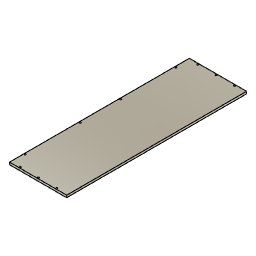
side_cover_lid v28 (Autodesk Fusion 360 design; units mm, degrees)
Autodesk Fusion 360 part; units mm, degrees
sketch "Sketch4" plane through (0, 0, 0) normal (1, 0, 0) x (0, 1, 0)
  line L0 (0, 0) -> (-450, 0)
  line L1 (-450, 0) -> (-450, 170.719)
  line L2 (-450, 170.719) -> (0, 170.719)
  line L3 (0, 170.719) -> (0, 0)
  dimension "d21" = 450
  dimension "d22" = 170.719
  constraint horizontal L0
  constraint vertical L1
  constraint horizontal L2
  constraint vertical L3
  constraint coincident L0.start L3.end
  measures "d21" distance of L0.start L0.end
  measures "d22" distance of L0.start L2.end
sketch "Sketch5" plane through (0, 0, 0) normal (-1, 0, 0) x (0, -1, 0)
  line L0 (450, 170.719) -> (0, 170.719)
  line L1 (0, 170.719) -> (0, 0)
  line L2 (0, 0) -> (450, 0)
  line L3 (450, 0) -> (450, 170.719)
  line L4 (0, 170.719) -> (455, 170.719)
  line L5 (455, 170.719) -> (455, 175.719)
  line L6 (455, 175.719) -> (0, 175.719)
  line L7 (0, 175.719) -> (0, 170.719)
  line L8 (455, 175.719) -> (450, 175.719)
  line L9 (450, 175.719) -> (450, 0)
  line L10 (450, 0) -> (455, 0)
  line L11 (455, 0) -> (455, 175.719)
  line L12 (0, 0) -> (-5, 0)
  line L13 (-5, 0) -> (-5, 175.719)
  line L14 (-5, 175.719) -> (0, 175.719)
  line L15 (0, 175.719) -> (0, 0)
  dimension "d25" = 455
  dimension "d26" = 5
  dimension "d27" = 5
  dimension "d28" = 175.719
  constraint horizontal L4
  constraint vertical L5
  constraint horizontal L6
  constraint vertical L7
  constraint coincident L0.end L1.start
  constraint horizontal L8
  constraint vertical L9
  constraint horizontal L10
  constraint vertical L11
  constraint coincident L2.end L3.start
  constraint horizontal L12
  constraint vertical L13
  constraint horizontal L14
  constraint vertical L15
  constraint coincident L1.end L2.start
  measures "d25" distance of L0.end L4.end
  measures "d26" distance of L0.end L6.end
  measures "d27" distance of L1.end L12.end
  measures "d28" distance of L1.end L6.end
extrude "Extrude7" add sketch "Sketch5" along normal blind 150 contours L3 L4 L9 L10 L11 | L0 L4 L6 L7 L9 L15 | L1 L7 L12 L13 L14 L15
extrude "Extrude8" add 1 faces at (-50, -451.6667, 170.719) along direction (0, 0, 1) blind 5
sketch "Sketch6" plane through (0, 0, 0) normal (1, 0, 0) x (0, 1, 0)
  line L0 (-450, 0) -> (-450, 170.719)
  line L1 (-450, 170.719) -> (0, 170.719)
  line L2 (0, 170.719) -> (0, 0)
  line L3 (0, 0) -> (5, 0)
  line L4 (5, 0) -> (5, 175.719)
  line L5 (5, 175.719) -> (-455, 175.719)
  line L6 (-455, 175.719) -> (-455, 0)
  line L7 (-455, 0) -> (-450, 0)
  line L8 (-455, 175.719) -> (5, 175.719)
  line L9 (5, 175.719) -> (5, 0)
  line L10 (5, 0) -> (-455, 0)
  line L11 (-455, 0) -> (-455, 175.719)
  constraint horizontal L8
  constraint vertical L9
  constraint horizontal L10
  constraint vertical L11
  constraint coincident L3.end L4.start
  constraint coincident L5.end L6.start
extrude "Extrude9" add sketch "Sketch6" along normal blind 5
sketch "Sketch7" plane through (0, -455, 0) normal (0, -1, 0) x (1, 0, 0)
  line L0 (5, 175.719) -> (-150, 175.719)
  line L1 (-150, 175.719) -> (-150, 0)
  line L2 (-150, 0) -> (5, 0)
  line L3 (5, 0) -> (5, 175.719)
  line L4 (-150, 0) -> (5, 0)
  line L5 (5, 0) -> (5, 5)
  line L6 (5, 5) -> (-150, 5)
  line L7 (-150, 5) -> (-150, 0)
  dimension "d35" = 5
  constraint horizontal L4
  constraint vertical L5
  constraint horizontal L6
  constraint vertical L7
  constraint coincident L3 L5.end
  constraint coincident L1.end L2.start
  measures "d35" distance of L1.end L6.end
extrude "Extrude10" add sketch "Sketch7" along normal blind 20 contours L1 L2 L3 L4 L5 L6 L7
sketch "Sketch8" plane through (0, 5, 0) normal (0, 1, 0) x (-1, 0, 0)
  line L0 (-5, 0) -> (150, 0)
  line L1 (150, 0) -> (150, 175.719)
  line L2 (150, 175.719) -> (-5, 175.719)
  line L3 (-5, 175.719) -> (-5, 0)
  line L4 (150, 0) -> (-5, 0)
  line L5 (-5, 0) -> (-5, 5)
  line L6 (-5, 5) -> (150, 5)
  line L7 (150, 5) -> (150, 0)
  dimension "d38" = 5
  constraint horizontal L4
  constraint vertical L5
  constraint horizontal L6
  constraint vertical L7
  constraint coincident L3 L5.end
  constraint coincident L0.end L1.start
  measures "d38" distance of L0.end L6.end
extrude "Extrude11" add sketch "Sketch8" along normal blind 20 contours L0 L1 L3 L4 L5 L6 L7
sketch "Sketch9" plane through (5, 0, 0) normal (1, 0, 0) x (0, 1, 0)
  line L0 (-475, 0) -> (25, 0)
  line L1 (25, 0) -> (25, 5)
  line L2 (25, 5) -> (5, 5)
  line L3 (5, 5) -> (5, 175.719)
  line L4 (5, 175.719) -> (-455, 175.719)
  line L5 (-455, 175.719) -> (-455, 5)
  line L6 (-455, 5) -> (-475, 5)
  line L7 (-475, 5) -> (-475, 0)
  line L8 (-475, 5) -> (25, 5)
  line L9 (25, 5) -> (25, 0)
  line L10 (25, 0) -> (-475, 0)
  line L11 (-475, 0) -> (-475, 5)
  constraint horizontal L8
  constraint vertical L9
  constraint horizontal L10
  constraint vertical L11
  constraint coincident L0.end L1.start
  constraint coincident L6.end L7.start
extrude "Extrude12" add sketch "Sketch9" along normal blind 20 contours L0 L1 L2 L6 L7 L8 L9 L10 L11
sketch "Sketch10" plane through (0, 0, 5) normal (0, 0, 1) x (-1, 0, 0)
  line L0 (150, -5) -> (-5, -5)
  line L1 (-5, -5) -> (-5, 455)
  line L2 (-5, 455) -> (150, 455)
  line L3 (150, 455) -> (150, 475)
  line L4 (150, 475) -> (-25, 475)
  line L5 (-25, 475) -> (-25, -25)
  line L6 (-25, -25) -> (150, -25)
  line L7 (150, -25) -> (150, -5)
  line L8 (-25, -25) -> (-5, -25)
  line L9 (-5, -25) -> (-5, -5)
  line L10 (-5, -5) -> (-25, -5)
  line L11 (-25, -5) -> (-25, -25)
  line L12 (-25, 475) -> (-5, 475)
  line L13 (-5, 475) -> (-5, 455)
  line L14 (-5, 455) -> (-25, 455)
  line L15 (-25, 455) -> (-25, 475)
  constraint horizontal L8
  constraint vertical L9
  constraint horizontal L10
  constraint vertical L11
  constraint coincident L0.end L1.start
  constraint coincident L5.end L6.start
  constraint horizontal L12
  constraint vertical L13
  constraint horizontal L14
  constraint vertical L15
  constraint coincident L1.end L2.start
  constraint coincident L4.end L5.start
extrude "Extrude13" cut sketch "Sketch10" against normal blind 50 contours L5 L6 L8 L9 L10 L11 | L4 L5 L12 L13 L14 L15
sketch "Sketch11" plane through (0, 0, 5) normal (0, 0, 1) x (-1, 0, 0)
  line L0 (-5, 475) -> (-5, 455)
  line L1 (-5, 455) -> (150, 455)
  line L2 (150, 455) -> (150, 475)
  line L3 (150, 475) -> (-5, 475)
  line L4 (-5, -25) -> (15, -25)
  line L5 (15, -25) -> (15, -15)
  line L6 (15, -15) -> (-5, -15)
  line L7 (-5, -15) -> (-5, -25)
  line L8 (150, -25) -> (130, -25)
  line L9 (130, -25) -> (130, -15)
  line L10 (130, -15) -> (150, -15)
  line L11 (150, -15) -> (150, -25)
  line L12 (130, -15) -> (72.5, -15)
  line L13 (150, 475) -> (130, 475)
  line L14 (130, 475) -> (130, 465)
  line L15 (130, 465) -> (150, 465)
  line L16 (150, 465) -> (150, 475)
  line L17 (-5, 475) -> (15, 475)
  line L18 (15, 475) -> (15, 465)
  line L19 (15, 465) -> (-5, 465)
  line L20 (-5, 465) -> (-5, 475)
  line L21 (130, 465) -> (72.5, 465)
  line L22 (-5, 455) -> (-15, 455)
  line L23 (-15, 455) -> (-15, 435)
  line L24 (-15, 435) -> (-5, 435)
  line L25 (-5, 435) -> (-5, 455)
  line L26 (-5, -5) -> (-15, -5)
  line L27 (-15, -5) -> (-15, 15)
  line L28 (-15, 15) -> (-5, 15)
  line L29 (-5, 15) -> (-5, -5)
  line L30 (-15, 15) -> (-15, 99)
  line L31 (-15, 99) -> (-15, 183)
  line L32 (-15, 183) -> (-15, 267)
  line L33 (-15, 267) -> (-15, 351)
  line L34 (-15, 351) -> (-15, 435)
  dimension "d45" = 20
  dimension "d46" = 10
  dimension "d47" = 20
  dimension "d48" = 10
  dimension "d49" = 57.5
  dimension "d50" = 20
  dimension "d51" = 20
  dimension "d52" = 57.5
  dimension "d53" = 10
  dimension "d54" = 20
  dimension "d55" = 10
  dimension "d56" = 20
  dimension "d57" = 84
  dimension "d58" = 84
  dimension "d59" = 84
  dimension "d60" = 84
  dimension "d61" = 84
  constraint horizontal L4
  constraint vertical L5
  constraint horizontal L6
  constraint vertical L7
  constraint horizontal L8
  constraint vertical L9
  constraint horizontal L10
  constraint vertical L11
  constraint perpendicular L9 L12
  constraint horizontal L13
  constraint vertical L14
  constraint horizontal L15
  constraint vertical L16
  constraint coincident L2.end L3.start
  constraint horizontal L17
  constraint vertical L18
  constraint horizontal L19
  constraint vertical L20
  constraint coincident L0.start L3.end
  constraint perpendicular L14 L21
  constraint horizontal L22
  constraint vertical L23
  constraint horizontal L24
  constraint vertical L25
  constraint coincident L0.end L1.start
  constraint horizontal L26
  constraint vertical L27
  constraint horizontal L28
  constraint vertical L29
  constraint perpendicular L28 L30
  constraint parallel L30 L31
  constraint parallel L31 L32
  constraint parallel L32 L33
  constraint vertical L34
  measures "d45" distance of L4.start L4.end
  measures "d46" distance of L4.start L6.end
  measures "d47" distance of L8.start L8.end
  measures "d48" distance of L8.start L10.end
  measures "d49" distance of L9.end L12.end
  measures "d50" distance of L2.end L13.end
  measures "d51" distance of L0.start L17.end
  measures "d52" distance of L14.end L21.end
  measures "d53" distance of L0.end L22.end
  measures "d54" distance of L0.end L24.end
  measures "d55" distance of L26.start L26.end
  measures "d56" distance of L26.start L28.end
  measures "d57" distance of L27.end L30.end
  measures "d58" distance of L30.end L31.end
  measures "d59" distance of L31.end L32.end
  measures "d60" distance of L32.end L33.end
  measures "d61" distance of L33.end L23.end
hole "Hole1" at (-130, -465, 5) at (-72.5, -465, 5) at (-15, -465, 5) at (15, -435, 5) at (15, -351, 5) at (15, -267, 5) at (15, -183, 5) at (15, -99, 5) at (15, -15, 5) at (-15, 15, 5) at (-72.5, 15, 5) at (-130, 15, 5) direction (0, 0, -1) diameter 7.035 depth 10 tip angle 180
thread "Thread1" "ISO Metric profile 8.0 M8x1 6H"
extrude "Extrude14" add 1 faces at (-98.3333, -148.3333, 175.719) along direction (0, 0, 1) blind 5
extrude "Extrude15" add 1 faces at (-46.6667, 5, 122.146) along direction (0, 1, 0) blind 5
extrude "Extrude16" add 1 faces at (-46.6667, -455, 122.146) along direction (0, -1, 0) blind 5
extrude "Extrude17" add 1 faces at (-144.4764, -463.0724, 0) along direction (0, 0, -1) blind 5
extrude "Extrude18" add 1 faces at (-46.6667, 25, -1.6667) along direction (0, 1, 0) blind 5
extrude "Extrude19" add 1 faces at (-46.6667, -475, -1.6667) along direction (0, -1, 0) blind 5
extrude "Extrude20" add 1 faces at (25, -301.6667, 1.6667) along direction (1, 0, 0) blind 5
extrude "Extrude21" add 1 faces at (21.6667, -455, 1.6667) along direction (0, -1, 0) blind 25
extrude "Extrude22" add 1 faces at (21.6667, 5, 1.6667) along direction (0, 1, 0) blind 25
sketch "Sketch12" plane through (0, 0, 5) normal (0, 0, 1) x (-1, 0, 0)
  circle A0 centre (72.5, 465) radius 3.5175
  circle A1 centre (130, 465) radius 3.5175
  circle A2 centre (15, 465) radius 3.5175
  circle A3 centre (-15, 15) radius 3.5175
  circle A4 centre (-15, 183) radius 3.5175
  circle A5 centre (-15, 351) radius 3.5175
  circle A6 centre (-15, 435) radius 3.5175
  circle A7 centre (-15, 267) radius 3.5175
  circle A8 centre (-15, 99) radius 3.5175
  line L0 (150, -10) -> (-5, -10)
  line L1 (-5, -10) -> (-5, 460)
  line L2 (-5, 460) -> (150, 460)
  line L3 (150, 460) -> (150, 480)
  line L4 (150, 480) -> (-30, 480)
  line L5 (-30, 480) -> (-30, -30)
  line L6 (-30, -30) -> (150, -30)
  line L7 (150, -30) -> (150, -10)
  circle A9 centre (72.5, -15) radius 3.5175
  circle A10 centre (15, -15) radius 3.5175
  circle A11 centre (130, -15) radius 3.5175
  line L8 (130, -15) -> (130, -20)
  line L9 (130, 465) -> (130, 470)
  line L10 (72.5, 465) -> (72.5, 470)
  line L11 (15, 465) -> (15, 470)
  line L12 (-15, 435) -> (-20, 435)
  line L13 (-15, 351) -> (-20, 351)
  line L14 (-15, 267) -> (-20, 267)
  line L15 (-15, 183) -> (-20, 183)
  line L16 (72.5, -15) -> (72.5, -20)
  line L17 (15, -15) -> (15, -20)
  line L18 (-15, 15) -> (-20, 15)
  line L19 (-15, 99) -> (-20, 99)
  dimension "d83" = 5
  dimension "d84" = 5
  dimension "d85" = 5
  dimension "d86" = 5
  dimension "d87" = 5
  dimension "d88" = 5
  dimension "d89" = 5
  dimension "d90" = 5
  dimension "d91" = 5
  dimension "d92" = 5
  dimension "d93" = 5
  dimension "d94" = 5
  constraint coincident A11.centre L8.start
  constraint perpendicular L6 L8
  constraint coincident A1.centre L9.start
  constraint perpendicular L2 L9
  constraint coincident A0.centre L10.start
  constraint perpendicular L2 L10
  constraint coincident A2.centre L11.start
  constraint perpendicular L4 L11
  constraint coincident A6.centre L12.start
  constraint horizontal L12
  constraint coincident A5.centre L13.start
  constraint perpendicular L5 L13
  constraint coincident A7.centre L14.start
  constraint perpendicular L1 L14
  constraint coincident A4.centre L15.start
  constraint perpendicular L1 L15
  constraint coincident A9.centre L16.start
  constraint perpendicular L0 L16
  constraint coincident A10.centre L17.start
  constraint perpendicular L0 L17
  constraint coincident A3.centre L18.start
  constraint horizontal L18
  constraint coincident A8.centre L19.start
  constraint perpendicular L5 L19
  measures "d83" distance of A11.centre L8.end
  measures "d84" distance of A1.centre L9.end
  measures "d85" distance of A0.centre L10.end
  measures "d86" distance of A2.centre L11.end
  measures "d87" distance of A6.centre L12.end
  measures "d88" distance of A5.centre L13.end
  measures "d89" distance of A7.centre L14.end
  measures "d90" distance of A4.centre L15.end
  measures "d91" distance of A9.centre L16.end
  measures "d92" distance of A10.centre L17.end
  measures "d93" distance of A3.centre L18.end
  measures "d94" distance of A8.centre L19.end
delete_face "DeleteFace1" 1 faces at (15.1753, -18.5131, -1.6667)
delete_face "DeleteFace2" 1 faces at (-14.8247, 11.4869, -1.6667)
delete_face "DeleteFace3" 1 faces at (-71.2969, 18.3054, -1.6667)
delete_face "DeleteFace4" 1 faces at (-129.8247, 11.4869, -1.6667)
delete_face "DeleteFace5" 1 faces at (15.1753, -102.5131, -1.6667)
delete_face "DeleteFace6" 1 faces at (-133.5164, -464.9123, -1.6667)
delete_face "DeleteFace7" 1 faces at (-76.0164, -464.9123, -1.6667)
delete_face "DeleteFace8" 1 faces at (-18.5164, -464.9123, -1.6667)
delete_face "DeleteFace9" 1 faces at (11.4836, -434.9123, -1.6667)
delete_face "DeleteFace10" 1 faces at (11.4836, -350.9123, -1.6667)
delete_face "DeleteFace11" 1 faces at (11.4836, -266.9123, -1.6667)
delete_face "DeleteFace12" 1 faces at (17.261, -180.3054, -1.6667)
hole "Hole2" at (-130, 20, 5) at (-72.5, 20, 5) at (-15, 20, 5) at (20, -15, 5) at (20, -99, 5) at (20, -183, 5) at (20, -267, 5) at (20, -351, 5) at (20, -435, 5) at (-15, -470, 5) at (-72.5, -470, 5) at (-130, -470, 5) direction (0, 0, -1) diameter 7.035 depth 38 tip angle 180
thread "Thread2" "ISO Metric profile 8.0 M8x1 6H"
extrude "Extrude23" add 1 faces at (-50, -300, 170.719) along direction (0, 0, -1) blind 43
extrude "Extrude24" cut 1 faces at (-98.3333, -303.3333, 180.719) along direction (0, 0, -1) blind 43
extrude "Extrude25" cut 1 faces at (30, -140, -1.6667) along direction (-1, 0, 0) blind 5
sketch "Sketch13" plane through (0, 0, 5) normal (0, 0, 1) x (-1, 0, 0)
  line L0 (-25, 480) -> (-25, -30)
  line L1 (-25, -30) -> (150, -30)
  line L2 (150, -30) -> (150, -10)
  line L3 (150, -10) -> (-5, -10)
  line L4 (-5, -10) -> (-5, 460)
  line L5 (-5, 460) -> (150, 460)
  line L6 (150, 460) -> (150, 480)
  line L7 (150, 480) -> (-25, 480)
  circle A0 centre (72.5, 470) radius 3.5175
  circle A1 centre (-20, 435) radius 3.5175
  circle A2 centre (-20, 267) radius 3.5175
  circle A3 centre (-20, 99) radius 3.5175
  circle A4 centre (15, -20) radius 3.5175
  circle A5 centre (130, -20) radius 3.5175
  circle A6 centre (72.5, -20) radius 3.5175
  circle A7 centre (-20, 15) radius 3.5175
  circle A8 centre (-20, 183) radius 3.5175
  circle A9 centre (-20, 351) radius 3.5175
  circle A10 centre (15, 470) radius 3.5175
  circle A11 centre (130, 470) radius 3.5175
  line L8 (-20, 435) -> (-15, 435)
  line L9 (-20, 351) -> (-15, 351)
  line L10 (-20, 267) -> (-15, 267)
  line L11 (-20, 183) -> (-15, 183)
  line L12 (-20, 99) -> (-15, 99)
  dimension "d104" = 5
  dimension "d105" = 5
  dimension "d106" = 5
  dimension "d107" = 5
  dimension "d108" = 5
  constraint coincident A1.centre L8.start
  constraint horizontal L8
  constraint coincident A9.centre L9.start
  constraint perpendicular L0 L9
  constraint coincident A2.centre L10.start
  constraint perpendicular L0 L10
  constraint coincident A8.centre L11.start
  constraint perpendicular L4 L11
  constraint coincident A3.centre L12.start
  constraint perpendicular L4 L12
  measures "d104" distance of A1.centre L8.end
  measures "d105" distance of A9.centre L9.end
  measures "d106" distance of A2.centre L10.end
  measures "d107" distance of A8.centre L11.end
  measures "d108" distance of A3.centre L12.end
delete_face "DeleteFace13" 1 faces at (16.4836, -434.9123, 1.6667)
delete_face "DeleteFace14" 1 faces at (16.4836, -350.9123, 1.6667)
delete_face "DeleteFace15" 1 faces at (22.261, -180.3054, 1.6667)
delete_face "DeleteFace16" 1 faces at (16.4836, -266.9123, 1.6667)
sketch "Sketch14" plane through (0, 0, 5) normal (0, 0, 1) x (-1, 0, 0)
  line L0 (-20, 15) -> (-15, 15)
  dimension "d109" = 5
  constraint horizontal L0
  measures "d109" distance of L0.start L0.end
delete_face "DeleteFace17" 1 faces at (20.1753, -18.5131, 1.6667)
delete_face "DeleteFace18" 1 faces at (20.1753, -102.5131, 1.6667)
extrude "Extrude26" cut 1 faces at (-50, -300, 127.719) along direction (0, 0, 1) blind 5
extrude "Extrude27" add 1 faces at (-98.3333, -303.3333, 137.719) along direction (0, 0, 1) blind 5
extrude "Extrude28" add 1 faces at (0, -150, 86.8127) along direction (-1, 0, 0) blind 5
extrude "Extrude29" cut 1 faces at (-5, -150, 86.8127) along direction (1, 0, 0) blind 5
extrude "Extrude30" add 1 faces at (5, -303.3333, 50.9063) along direction (1, 0, 0) blind 5
extrude "Extrude31" add 1 faces at (25, -140, -1.6667) along direction (1, 0, 0) blind 5
sketch "Sketch15" plane through (0, 0, 5) normal (0, 0, 1) x (-1, 0, 0)
  line L0 (-10, 460) -> (150, 460)
  line L1 (150, 460) -> (150, 480)
  line L2 (150, 480) -> (-30, 480)
  line L3 (-30, 480) -> (-30, -30)
  line L4 (-30, -30) -> (150, -30)
  line L5 (150, -30) -> (150, -10)
  line L6 (150, -10) -> (-10, -10)
  line L7 (-10, -10) -> (-10, 460)
  circle A0 centre (72.5, 470) radius 3.5175
  circle A1 centre (15, -20) radius 3.5175
  circle A2 centre (130, -20) radius 3.5175
  circle A3 centre (72.5, -20) radius 3.5175
  circle A4 centre (15, 470) radius 3.5175
  circle A5 centre (130, 470) radius 3.5175
  line L8 (-15, 435) -> (-20, 435)
  line L9 (-20, 435) -> (-20, 351)
  line L10 (-20, 351) -> (-20, 267)
  line L11 (-20, 267) -> (-20, 183)
  line L12 (-20, 183) -> (-20, 99)
  line L13 (-20, 99) -> (-20, 15)
  dimension "d125" = 5
  dimension "d126" = 84
  dimension "d127" = 84
  dimension "d128" = 84
  dimension "d129" = 84
  constraint perpendicular L3 L8
  constraint perpendicular L8 L9
  constraint perpendicular L8 L10
  constraint parallel L7 L11
  constraint parallel L3 L12
  constraint parallel L3 L13
  measures "d125" distance of L8.start L8.end
  measures "d126" distance of L8.end L9.end
  measures "d127" distance of L9.end L10.end
  measures "d128" distance of L11.end L12.end
  measures "d129" distance of L12.end L13.end
hole "Hole4" at (20, -435, 5) at (20, -351, 5) at (20, -267, 5) at (20, -183, 5) at (20, -15, 5) at (20, -99, 5) direction (0, 0, -1) diameter 7.035 depth 50 tip angle 180
thread "Thread4" "ISO Metric profile 8.0 M8x1 6H"
extrude "Extrude32" cut 1 faces at (-90, -480, -1.6667) along direction (0, 1, 0) blind 20
extrude "Extrude33" cut 1 faces at (30, -296.6667, -1.6667) along direction (-1, 0, 0) blind 20
extrude "Extrude34" cut 1 faces at (-96.6667, 30, -1.6667) along direction (0, -1, 0) blind 20
extrude "Extrude35" cut 1 faces at (6.6667, -150, -5) along direction (0, 0, 1) blind 137.19
extrude "Extrude36" cut 1 faces at (6.6667, -150, 132.19) along direction (0, 0, 1) blind 0.529
sketch "Sketch16" plane through (0, 0, 142.719) normal (0, 0, 1) x (-1, 0, 0)
  line L0 (150, -10) -> (150, 460)
  line L1 (150, 460) -> (-10, 460)
  line L2 (-10, 460) -> (-10, -10)
  line L3 (-10, -10) -> (150, -10)
  line L4 (150, -10) -> (125, -10)
  line L5 (125, -10) -> (125, -5)
  line L6 (125, -5) -> (150, -5)
  line L7 (150, -5) -> (150, -10)
  line L8 (-10, -10) -> (15, -10)
  line L9 (15, -10) -> (15, -5)
  line L10 (15, -5) -> (-10, -5)
  line L11 (-10, -5) -> (-10, -10)
  line L12 (150, 460) -> (125, 460)
  line L13 (125, 460) -> (125, 455)
  line L14 (125, 455) -> (150, 455)
  line L15 (150, 455) -> (150, 460)
  line L16 (-10, 460) -> (15, 460)
  line L17 (15, 460) -> (15, 455)
  line L18 (15, 455) -> (-10, 455)
  line L19 (-10, 455) -> (-10, 460)
  dimension "d143" = 25
  dimension "d144" = 5
  dimension "d145" = 25
  dimension "d146" = 5
  dimension "d147" = 25
  dimension "d148" = 5
  dimension "d149" = 25
  dimension "d150" = 5
  constraint horizontal L4
  constraint vertical L5
  constraint horizontal L6
  constraint vertical L7
  constraint coincident L0.start L3.end
  constraint horizontal L8
  constraint vertical L9
  constraint horizontal L10
  constraint vertical L11
  constraint coincident L2.end L3.start
  constraint horizontal L12
  constraint vertical L13
  constraint horizontal L14
  constraint vertical L15
  constraint coincident L0.end L1.start
  constraint horizontal L16
  constraint vertical L17
  constraint horizontal L18
  constraint vertical L19
  constraint coincident L1.end L2.start
  measures "d143" distance of L0.start L4.end
  measures "d144" distance of L0.start L6.end
  measures "d145" distance of L2.end L8.end
  measures "d146" distance of L2.end L10.end
  measures "d147" distance of L0.end L12.end
  measures "d148" distance of L0.end L14.end
  measures "d149" distance of L1.end L16.end
  measures "d150" distance of L1.end L18.end
hole "Hole5" at (-125, -455, 142.719) at (-15, -455, 142.719) at (-15, 5, 142.719) at (-125, 5, 142.719) direction (0, 0, -1) diameter 6.78 depth 10 tip angle 180
sketch "Sketch17" plane through (0, 0, 142.719) normal (0, 0, 1) x (-1, 0, 0)
  circle A0 centre (15, -5) radius 3.39
  circle A1 centre (125, 455) radius 3.39
  circle A2 centre (15, 455) radius 3.39
  circle A3 centre (125, -5) radius 3.39
  line L0 (150, -10) -> (150, 460)
  line L1 (150, 460) -> (-10, 460)
  line L2 (-10, 460) -> (-10, -10)
  line L3 (-10, -10) -> (150, -10)
  line L4 (150, -10) -> (145, -10)
  line L5 (145, -10) -> (145, 225)
  line L6 (145, 225) -> (150, 225)
  line L7 (150, 225) -> (150, -10)
  line L8 (150, -10) -> (145, -10)
  line L9 (145, -10) -> (145, 50)
  line L10 (145, 50) -> (150, 50)
  line L11 (150, 50) -> (150, -10)
  line L12 (150, 460) -> (145, 460)
  line L13 (145, 460) -> (145, 400)
  line L14 (145, 400) -> (150, 400)
  line L15 (150, 400) -> (150, 460)
  dimension "d154" = 5
  dimension "d155" = 235
  dimension "d156" = 60
  dimension "d157" = 5
  dimension "d158" = 60
  constraint horizontal L4
  constraint vertical L5
  constraint horizontal L6
  constraint vertical L7
  constraint coincident L0.start L3.end
  constraint horizontal L8
  constraint vertical L9
  constraint horizontal L10
  constraint vertical L11
  constraint horizontal L12
  constraint vertical L13
  constraint horizontal L14
  constraint vertical L15
  constraint coincident L0.end L1.start
  measures "d154" distance of L0.start L4.end
  measures "d155" distance of L0.start L6.end
  measures "d156" distance of L0.start L10.end
  measures "d157" distance of L0.end L12.end
  measures "d158" distance of L0.end L14.end
sketch "Sketch18" plane through (0, 0, 142.719) normal (0, 0, 1) x (-1, 0, 0)
  circle A0 centre (15, -5) radius 3.39
  circle A1 centre (125, 455) radius 3.39
  circle A2 centre (15, 455) radius 3.39
  circle A3 centre (125, -5) radius 3.39
  line L0 (150, -10) -> (150, 460)
  line L1 (150, 460) -> (-10, 460)
  line L2 (-10, 460) -> (-10, -10)
  line L3 (-10, -10) -> (150, -10)
  line L4 (125, 455) -> (115, 455)
  line L5 (125, -5) -> (115, -5)
  dimension "d162" = 10
  dimension "d163" = 10
  constraint coincident A1.centre L4.start
  constraint parallel L1 L4
  constraint horizontal L5
  constraint coincident A3.centre L5.start
  measures "d162" distance of A1.centre L4.end
  measures "d163" distance of A3.centre L5.end
hole "Hole7" at (-115, 5, 142.719) at (-115, -455, 142.719) direction (0, 0, -1) diameter 6.78 depth 60 tip angle 180
delete_face "DeleteFace19" 1 faces at (-128.3889, -454.9155, 139.3857)
delete_face "DeleteFace20" 1 faces at (-127.7525, 6.9789, 139.3857)
extrude "Extrude37" cut 1 faces at (-48.6517, -300.5824, 142.719) along direction (0, 0, -1) blind 4
extrude "Extrude38" cut 1 faces at (-43.3333, -460, 134.719) along direction (0, 1, 0) blind 4
extrude "Extrude39" cut 1 faces at (-43.3333, 10, 134.719) along direction (0, -1, 0) blind 4
extrude "Extrude40" cut 1 faces at (10, -148, 136.719) along direction (-1, 0, 0) blind 4
delete_face "DeleteFace21" 1 faces at (-18.285, 5.8373, 136.719)
delete_face "DeleteFace22" 1 faces at (-114.9155, 1.6111, 136.719)
delete_face "DeleteFace23" 1 faces at (-118.3858, -455.1697, 136.719)
delete_face "DeleteFace24" 1 faces at (-18.3858, -455.1697, 136.719)
sketch "Sketch19" plane through (0, 0, 138.719) normal (0, 0, 1) x (-1, 0, 0)
  line L0 (150, 456) -> (-6, 456)
  line L1 (-6, 456) -> (-6, -6)
  line L2 (-6, -6) -> (150, -6)
  line L3 (150, -6) -> (150, 456)
  line L4 (150, -6) -> (119, -6)
  line L5 (119, -6) -> (119, -3)
  line L6 (119, -3) -> (150, -3)
  line L7 (150, -3) -> (150, -6)
  line L8 (-6, -6) -> (19, -6)
  line L9 (19, -6) -> (19, -3)
  line L10 (19, -3) -> (-6, -3)
  line L11 (-6, -3) -> (-6, -6)
  line L12 (150, 456) -> (119, 456)
  line L13 (119, 456) -> (119, 453)
  line L14 (119, 453) -> (150, 453)
  line L15 (150, 453) -> (150, 456)
  dimension "d175" = 31
  dimension "d176" = 3
  dimension "d177" = 25
  dimension "d178" = 3
  dimension "d179" = 31
  dimension "d180" = 3
  constraint horizontal L4
  constraint vertical L5
  constraint horizontal L6
  constraint vertical L7
  constraint coincident L2.end L3.start
  constraint horizontal L8
  constraint vertical L9
  constraint horizontal L10
  constraint vertical L11
  constraint coincident L1.end L2.start
  constraint horizontal L12
  constraint vertical L13
  constraint horizontal L14
  constraint vertical L15
  constraint coincident L0.start L3.end
  measures "d175" distance of L2.end L4.end
  measures "d176" distance of L2.end L6.end
  measures "d177" distance of L1.end L8.end
  measures "d178" distance of L1.end L10.end
  measures "d179" distance of L0.start L12.end
  measures "d180" distance of L0.start L14.end
sketch "Sketch20" plane through (0, 0, 138.719) normal (0, 0, 1) x (-1, 0, 0)
  line L0 (-6.316, 455.8332) -> (18.684, 455.8332)
  line L1 (18.684, 455.8332) -> (18.684, 452.8332)
  line L2 (18.684, 452.8332) -> (-6.316, 452.8332)
  line L3 (-6.316, 452.8332) -> (-6.316, 455.8332)
  dimension "d181" = 25
  dimension "d182" = 3
  constraint horizontal L0
  constraint vertical L1
  constraint horizontal L2
  constraint vertical L3
  measures "d181" distance of L0.start L0.end
  measures "d182" distance of L0.start L2.end
sketch "Sketch21" plane through (0, 0, 138.719) normal (0, 0, 1) x (-1, 0, 0)
  line L0 (150, 456) -> (-6, 456)
  line L1 (-6, 456) -> (-6, -6)
  line L2 (-6, -6) -> (150, -6)
  line L3 (150, -6) -> (150, 456)
  line L4 (-6, 456) -> (-3, 456)
  line L5 (-3, 456) -> (-3, 396)
  line L6 (-3, 396) -> (-6, 396)
  line L7 (-6, 396) -> (-6, 456)
  line L8 (-6, -6) -> (-3, -6)
  line L9 (-3, -6) -> (-3, 54)
  line L10 (-3, 54) -> (-6, 54)
  line L11 (-6, 54) -> (-6, -6)
  line L12 (-3, 396) -> (-3, 225)
  dimension "d186" = 3
  dimension "d187" = 60
  dimension "d188" = 3
  dimension "d189" = 60
  constraint horizontal L4
  constraint vertical L5
  constraint horizontal L6
  constraint vertical L7
  constraint coincident L0.end L1.start
  constraint horizontal L8
  constraint vertical L9
  constraint horizontal L10
  constraint vertical L11
  constraint coincident L1.end L2.start
  constraint perpendicular L6 L12
  measures "d186" distance of L0.end L4.end
  measures "d187" distance of L0.end L6.end
  measures "d188" distance of L1.end L8.end
  measures "d189" distance of L1.end L10.end
sketch "Sketch22" plane through (0, 0, 138.719) normal (0, 0, 1) x (-1, 0, 0)
  line L0 (150, 456) -> (-6, 456)
  line L1 (-6, 456) -> (-6, -6)
  line L2 (-6, -6) -> (150, -6)
  line L3 (150, -6) -> (150, 456)
  line L4 (150, -6) -> (147, -6)
  line L5 (147, -6) -> (147, 54)
  line L6 (147, 54) -> (150, 54)
  line L7 (150, 54) -> (150, -6)
  line L8 (150, 456) -> (147, 456)
  line L9 (147, 456) -> (147, 396)
  line L10 (147, 396) -> (150, 396)
  line L11 (150, 396) -> (150, 456)
  line L12 (147, 396) -> (147, 225)
  dimension "d193" = 3
  dimension "d194" = 60
  dimension "d195" = 3
  dimension "d196" = 60
  constraint horizontal L4
  constraint vertical L5
  constraint horizontal L6
  constraint vertical L7
  constraint coincident L2.end L3.start
  constraint horizontal L8
  constraint vertical L9
  constraint horizontal L10
  constraint vertical L11
  constraint coincident L0.start L3.end
  constraint perpendicular L10 L12
  measures "d193" distance of L2.end L4.end
  measures "d194" distance of L2.end L6.end
  measures "d195" distance of L0.start L8.end
  measures "d196" distance of L0.start L10.end
sketch "Sketch23" plane through (0, 0, 138.719) normal (0, 0, 1) x (-1, 0, 0)
  line L0 (150, 456) -> (-6, 456)
  line L1 (-6, 456) -> (-6, -6)
  line L2 (-6, -6) -> (150, -6)
  line L3 (150, -6) -> (150, 456)
  line L4 (119, 453) -> (19, 453)
  dimension "d200" = 100
  constraint horizontal L4
  measures "d200" distance of L4.start L4.end
extrude "Extrude41" add 1 faces at (-46, 6, 136.719) along direction (0, 1, 0) blind 0.502
sketch "Sketch24" plane through (0, 0, 138.719) normal (0, 0, 1) x (-1, 0, 0)
  line L0 (150, 456) -> (-6, 456)
  line L1 (-6, 456) -> (-6, -6.502)
  line L2 (-6, -6.502) -> (150, -6.502)
  line L3 (150, -6.502) -> (150, 456)
  line L4 (150, -6.502) -> (119, -6.502)
  line L5 (119, -6.502) -> (119, -3.502)
  line L6 (119, -3.502) -> (150, -3.502)
  line L7 (150, -3.502) -> (150, -6.502)
  line L8 (-6, -6.502) -> (19, -6.502)
  line L9 (19, -6.502) -> (19, -3.502)
  line L10 (19, -3.502) -> (-6, -3.502)
  line L11 (-6, -3.502) -> (-6, -6.502)
  dimension "d206" = 31
  dimension "d207" = 3
  dimension "d208" = 25
  dimension "d209" = 3
  constraint horizontal L4
  constraint vertical L5
  constraint horizontal L6
  constraint vertical L7
  constraint coincident L2.end L3.start
  constraint horizontal L8
  constraint vertical L9
  constraint horizontal L10
  constraint vertical L11
  constraint coincident L1.end L2.start
  measures "d206" distance of L2.end L4.end
  measures "d207" distance of L2.end L6.end
  measures "d208" distance of L1.end L8.end
  measures "d209" distance of L1.end L10.end
sketch "Sketch25" plane through (0, 0, 138.719) normal (0, 0, 1) x (-1, 0, 0)
  line L0 (150, 456) -> (-6, 456)
  line L1 (-6, 456) -> (-6, -6.502)
  line L2 (-6, -6.502) -> (150, -6.502)
  line L3 (150, -6.502) -> (150, 456)
  line L4 (150, -6.502) -> (147, -6.502)
  line L5 (147, -6.502) -> (147, 53.498)
  line L6 (147, 53.498) -> (150, 53.498)
  line L7 (150, 53.498) -> (150, -6.502)
  dimension "d213" = 3
  dimension "d214" = 60
  constraint horizontal L4
  constraint vertical L5
  constraint horizontal L6
  constraint vertical L7
  constraint coincident L2.end L3.start
  measures "d213" distance of L2.end L4.end
  measures "d214" distance of L2.end L6.end
sketch "Sketch26" plane through (0, 0, 138.719) normal (0, 0, 1) x (-1, 0, 0)
  line L0 (150, 456) -> (-6, 456)
  line L1 (-6, 456) -> (-6, -6.502)
  line L2 (-6, -6.502) -> (150, -6.502)
  line L3 (150, -6.502) -> (150, 456)
  line L4 (147, 53.498) -> (147, 224.749)
  dimension "d218" = 171.251
  constraint parallel L3 L4
  measures "d218" distance of L4.start L4.end
sketch "Sketch27" plane through (0, 0, 138.719) normal (0, 0, 1) x (-1, 0, 0)
  line L0 (150, 456) -> (-6, 456)
  line L1 (-6, 456) -> (-6, -6.502)
  line L2 (-6, -6.502) -> (150, -6.502)
  line L3 (150, -6.502) -> (150, 456)
  line L4 (150, 456) -> (124, 456)
  line L5 (124, 456) -> (124, 453)
  line L6 (124, 453) -> (150, 453)
  line L7 (150, 453) -> (150, 456)
  line L8 (-6, 456) -> (14, 456)
  line L9 (14, 456) -> (14, 453)
  line L10 (14, 453) -> (-6, 453)
  line L11 (-6, 453) -> (-6, 456)
  line L12 (124, 453) -> (69, 453)
  line L13 (150, -6.502) -> (124, -6.502)
  line L14 (124, -6.502) -> (124, -3.502)
  line L15 (124, -3.502) -> (150, -3.502)
  line L16 (150, -3.502) -> (150, -6.502)
  line L17 (124, -3.502) -> (69, -3.502)
  line L18 (-6, -6.502) -> (14, -6.502)
  line L19 (14, -6.502) -> (14, -3.502)
  line L20 (14, -3.502) -> (-6, -3.502)
  line L21 (-6, -3.502) -> (-6, -6.502)
  dimension "d222" = 26
  dimension "d223" = 3
  dimension "d224" = 20
  dimension "d225" = 3
  dimension "d227" = 55
  dimension "d228" = 26
  dimension "d229" = 3
  dimension "d230" = 55
  dimension "d231" = 20
  dimension "d232" = 3
  constraint horizontal L4
  constraint vertical L5
  constraint horizontal L6
  constraint vertical L7
  constraint coincident L0.start L3.end
  constraint horizontal L8
  constraint vertical L9
  constraint horizontal L10
  constraint vertical L11
  constraint coincident L0.end L1.start
  constraint perpendicular L9 L12
  constraint horizontal L13
  constraint vertical L14
  constraint horizontal L15
  constraint vertical L16
  constraint coincident L2.end L3.start
  constraint perpendicular L14 L17
  constraint horizontal L18
  constraint vertical L19
  constraint horizontal L20
  constraint vertical L21
  constraint coincident L1.end L2.start
  measures "d222" distance of L0.start L4.end
  measures "d223" distance of L0.start L6.end
  measures "d224" distance of L0.end L8.end
  measures "d225" distance of L0.end L10.end
  measures "d227" distance of L5.end L12.end
  measures "d228" distance of L2.end L13.end
  measures "d229" distance of L2.end L15.end
  measures "d230" distance of L14.end L17.end
  measures "d231" distance of L1.end L18.end
  measures "d232" distance of L1.end L20.end
hole "Hole15" at (-124, 3.502, 138.719) at (-69, 3.502, 138.719) at (-14, 3.502, 138.719) at (-124, -453, 138.719) at (-69, -453, 138.719) at (-14, -453, 138.719) direction (0, 0, -1) diameter 4.5 depth 10 tip angle 180
sketch "Sketch28" plane through (0, 0, 138.719) normal (0, 0, 1) x (-1, 0, 0)
  circle A0 centre (69, 453) radius 2.25
  circle A1 centre (14, -3.502) radius 2.25
  circle A2 centre (124, -3.502) radius 2.25
  circle A3 centre (69, -3.502) radius 2.25
  circle A4 centre (124, 453) radius 2.25
  circle A5 centre (14, 453) radius 2.25
  line L0 (150, 456) -> (-6, 456)
  line L1 (-6, 456) -> (-6, -6.502)
  line L2 (-6, -6.502) -> (150, -6.502)
  line L3 (150, -6.502) -> (150, 456)
  line L4 (150, 456) -> (147, 456)
  line L5 (147, 456) -> (147, 436)
  line L6 (147, 436) -> (150, 436)
  line L7 (150, 436) -> (150, 456)
  line L8 (150, -6.502) -> (147, -6.502)
  line L9 (147, -6.502) -> (147, 13.498)
  line L10 (147, 13.498) -> (150, 13.498)
  line L11 (150, 13.498) -> (150, -6.502)
  line L12 (147, 13.498) -> (147, 163.498)
  line L13 (147, 436) -> (147, 286)
  dimension "d236" = 3
  dimension "d237" = 20
  dimension "d238" = 3
  dimension "d239" = 20
  dimension "d240" = 150
  dimension "d241" = 150
  constraint horizontal L4
  constraint vertical L5
  constraint horizontal L6
  constraint vertical L7
  constraint coincident L0.start L3.end
  constraint horizontal L8
  constraint vertical L9
  constraint horizontal L10
  constraint vertical L11
  constraint coincident L2.end L3.start
  constraint perpendicular L10 L12
  constraint perpendicular L6 L13
  measures "d236" distance of L0.start L4.end
  measures "d237" distance of L0.start L6.end
  measures "d238" distance of L2.end L8.end
  measures "d239" distance of L2.end L10.end
  measures "d240" distance of L9.end L12.end
  measures "d241" distance of L5.end L13.end
hole "Hole16" at (-147, -436, 138.719) at (-147, -286, 138.719) at (-147, -163.498, 138.719) at (-147, -13.498, 138.719) direction (0, 0, -1) diameter 4.5 depth 10 tip angle 180
delete_face "DeleteFace31" 1 faces at (-126.2325, -453.2798, 136.719)
delete_face "DeleteFace32" 1 faces at (-71.2325, -453.2798, 136.719)
delete_face "DeleteFace33" 1 faces at (-16.2325, -453.2798, 136.719)
delete_face "DeleteFace34" 1 faces at (-149.2325, -436.2798, 136.719)
delete_face "DeleteFace35" 1 faces at (-149.2325, -286.2798, 136.719)
extrude "Extrude42" add 1 faces at (-46, -456, 136.719) along direction (0, -1, 0) blind 28
sketch "Sketch29" plane through (0, 0, 138.719) normal (0, 0, 1) x (-1, 0, 0)
  circle A0 centre (147, 163.498) radius 2.25
  circle A1 centre (147, 13.498) radius 2.25
  circle A2 centre (14, -3.502) radius 2.25
  circle A3 centre (124, -3.502) radius 2.25
  circle A4 centre (69, -3.502) radius 2.25
  line L0 (-6, 484) -> (-6, -6.502)
  line L1 (-6, -6.502) -> (150, -6.502)
  line L2 (150, -6.502) -> (150, 484)
  line L3 (150, 484) -> (-6, 484)
  line L4 (150, 484) -> (147, 484)
  line L5 (147, 484) -> (147, 464)
  line L6 (147, 464) -> (150, 464)
  line L7 (150, 464) -> (150, 484)
  line L8 (147, 464) -> (147, 314)
  line L9 (150, 484) -> (124, 484)
  line L10 (124, 484) -> (124, 481)
  line L11 (124, 481) -> (150, 481)
  line L12 (150, 481) -> (150, 484)
  line L13 (124, 481) -> (69, 481)
  line L14 (69, 481) -> (14, 481)
  dimension "d247" = 3
  dimension "d248" = 20
  dimension "d249" = 150
  dimension "d250" = 26
  dimension "d251" = 3
  dimension "d252" = 55
  dimension "d253" = 55
  constraint horizontal L4
  constraint vertical L5
  constraint horizontal L6
  constraint vertical L7
  constraint coincident L2.end L3.start
  constraint perpendicular L6 L8
  constraint horizontal L9
  constraint vertical L10
  constraint horizontal L11
  constraint vertical L12
  constraint perpendicular L10 L13
  constraint parallel L13 L14
  measures "d247" distance of L2.end L4.end
  measures "d248" distance of L2.end L6.end
  measures "d249" distance of L5.end L8.end
  measures "d250" distance of L2.end L9.end
  measures "d251" distance of L2.end L11.end
  measures "d252" distance of L10.end L13.end
  measures "d253" distance of L13.end L14.end
hole "Hole17" at (-147, -314, 138.719) at (-147, -464, 138.719) at (-124, -481, 138.719) at (-69, -481, 138.719) at (-14, -481, 138.719) direction (0, 0, -1) diameter 4.5 depth 10 tip angle 180
delete_face "DeleteFace36" 1 faces at (-149.2325, -464.2798, 136.719)
delete_face "DeleteFace37" 1 faces at (-126.2325, -481.2798, 136.719)
delete_face "DeleteFace38" 1 faces at (-71.2325, -481.2798, 136.719)
delete_face "DeleteFace39" 1 faces at (-16.2325, -481.2798, 136.719)
delete_face "DeleteFace40" 1 faces at (-145.1731, -12.1846, 136.719)
delete_face "DeleteFace41" 1 faces at (-123.2305, 5.6163, 136.719)
delete_face "DeleteFace42" 1 faces at (-68.2305, 5.6163, 136.719)
delete_face "DeleteFace43" 1 faces at (-13.776, 1.2632, 134.719)
sketch "Sketch30" plane through (0, 0, 138.719) normal (0, 0, 1) x (-1, 0, 0)
  circle A0 centre (147, 314) radius 2.25
  circle A1 centre (147, 163.498) radius 2.25
  line L0 (-6, 484) -> (-6, -6.502)
  line L1 (-6, -6.502) -> (150, -6.502)
  line L2 (150, -6.502) -> (150, 484)
  line L3 (150, 484) -> (-6, 484)
  line L4 (150, -6.502) -> (147, -6.502)
  line L5 (147, -6.502) -> (147, 33.498)
  line L6 (147, 33.498) -> (150, 33.498)
  line L7 (150, 33.498) -> (150, -6.502)
  line L8 (150, -6.502) -> (124, -6.502)
  line L9 (124, -6.502) -> (124, -3.502)
  line L10 (124, -3.502) -> (150, -3.502)
  line L11 (150, -3.502) -> (150, -6.502)
  line L12 (124, -3.502) -> (74, -3.502)
  line L13 (74, -3.502) -> (24, -3.502)
  line L14 (150, 484) -> (147, 484)
  line L15 (147, 484) -> (147, 444)
  line L16 (147, 444) -> (150, 444)
  line L17 (150, 444) -> (150, 484)
  line L18 (150, 484) -> (124, 484)
  line L19 (124, 484) -> (124, 481)
  line L20 (124, 481) -> (150, 481)
  line L21 (150, 481) -> (150, 484)
  line L22 (124, 481) -> (74, 481)
  line L23 (74, 481) -> (24, 481)
  dimension "d257" = 3
  dimension "d258" = 40
  dimension "d259" = 26
  dimension "d260" = 3
  dimension "d261" = 50
  dimension "d262" = 50
  dimension "d263" = 3
  dimension "d264" = 40
  dimension "d265" = 26
  dimension "d266" = 3
  dimension "d267" = 50
  dimension "d268" = 50
  constraint horizontal L4
  constraint vertical L5
  constraint horizontal L6
  constraint vertical L7
  constraint coincident L1.end L2.start
  constraint horizontal L8
  constraint vertical L9
  constraint horizontal L10
  constraint vertical L11
  constraint perpendicular L9 L12
  constraint parallel L12 L13
  constraint horizontal L14
  constraint vertical L15
  constraint horizontal L16
  constraint vertical L17
  constraint coincident L2.end L3.start
  constraint horizontal L18
  constraint vertical L19
  constraint horizontal L20
  constraint vertical L21
  constraint perpendicular L19 L22
  constraint parallel L22 L23
  measures "d257" distance of L1.end L4.end
  measures "d258" distance of L1.end L6.end
  measures "d259" distance of L1.end L8.end
  measures "d260" distance of L1.end L10.end
  measures "d261" distance of L9.end L12.end
  measures "d262" distance of L12.end L13.end
  measures "d263" distance of L2.end L14.end
  measures "d264" distance of L2.end L16.end
  measures "d265" distance of L2.end L18.end
  measures "d266" distance of L2.end L20.end
  measures "d267" distance of L19.end L22.end
  measures "d268" distance of L22.end L23.end
hole "Hole18" at (-24, -481, 138.719) at (-74, -481, 138.719) at (-124, -481, 138.719) at (-147, -444, 138.719) at (-147, -33.498, 138.719) at (-124, 3.502, 138.719) at (-24, 3.502, 138.719) direction (0, 0, -1) diameter 4.5 depth 10 tip angle 180
delete_face "DeleteFace44" 1 faces at (-145.8268, -161.5781, 136.719)
delete_face "DeleteFace45" 1 faces at (-149.2325, -314.2798, 136.719)
sketch "Sketch31" plane through (0, 0, 138.719) normal (0, 0, 1) x (-1, 0, 0)
  circle A0 centre (124, -3.502) radius 2.25
  circle A1 centre (147, 444) radius 2.25
  circle A2 centre (74, 481) radius 2.25
  circle A3 centre (24, 481) radius 2.25
  circle A4 centre (124, 481) radius 2.25
  circle A5 centre (147, 33.498) radius 2.25
  circle A6 centre (24, -3.502) radius 2.25
  line L0 (-6, 484) -> (-6, -6.502)
  line L1 (-6, -6.502) -> (150, -6.502)
  line L2 (150, -6.502) -> (150, 484)
  line L3 (150, 484) -> (-6, 484)
  line L4 (147, 444) -> (147, 294)
  line L5 (147, 33.498) -> (147, 183.498)
  dimension "d272" = 150
  dimension "d273" = 150
  constraint coincident A1.centre L4.start
  constraint parallel L2 L4
  constraint coincident A5.centre L5.start
  constraint parallel L2 L5
  measures "d272" distance of A1.centre L4.end
  measures "d273" distance of A5.centre L5.end
hole "Hole19" at (-147, -294, 138.719) at (-147, -444, 138.719) at (-147, -183.498, 138.719) at (-147, -33.498, 138.719) direction (0, 0, -1) diameter 4.5 depth 10 tip angle 180
sketch "Sketch32" plane through (0, 0, 138.719) normal (0, 0, 1) x (-1, 0, 0)
  circle A0 centre (147, 183.498) radius 2.25
  circle A1 centre (147, 294) radius 2.25
  circle A2 centre (124, -3.502) radius 2.25
  circle A3 centre (147, 444) radius 2.25
  circle A4 centre (74, 481) radius 2.25
  circle A5 centre (24, 481) radius 2.25
  circle A6 centre (124, 481) radius 2.25
  circle A7 centre (147, 33.498) radius 2.25
  circle A8 centre (24, -3.502) radius 2.25
  line L0 (-6, 484) -> (-6, -6.502)
  line L1 (-6, -6.502) -> (150, -6.502)
  line L2 (150, -6.502) -> (150, 484)
  line L3 (150, 484) -> (-6, 484)
  line L4 (24, -3.502) -> (74, -3.502)
  dimension "d277" = 50
  constraint coincident A8.centre L4.start
  constraint parallel L1 L4
  measures "d277" distance of A8.centre L4.end
hole "Hole20" at (-74, 3.502, 138.719) direction (0, 0, -1) diameter 4.5 depth 10 tip angle 180
equation "d49 = ( 115 / 2 ) * 1 mm"
equation "d52 = ( 115 / 2 ) * 1 mm"
equation "d155 = ( 470 / 2 ) * 1 mm"
equation "d218 = ( 342.502 / 2 ) * 1 mm"
